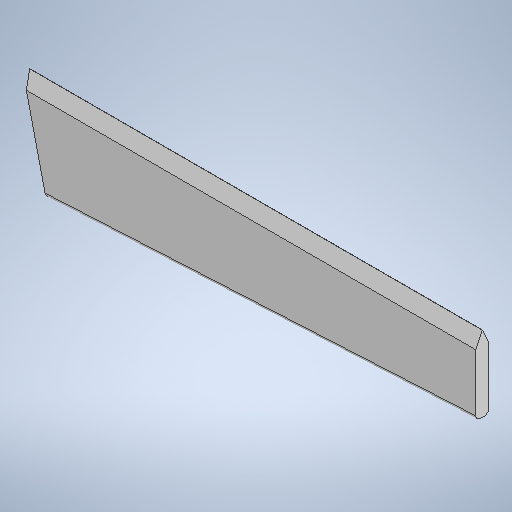
# Autodesk Inventor part: Part12
Saved by Autodesk Inventor 2025.3 (Build 293356000, 356)
## iProperties
Created: 2025-07-09
Part Number: Part12
Material: Generic
Document SubType Name: Modeling
Designer: steve
Density: 1 g/cm^3
Appearance: Default
Author: steve
Autodesk Inventor part; units mm, degrees
ref_plane "YZ Plane" through (0, 0, 0) normal (1, 0, 0) x (0, 1, 0)
ref_plane "XZ Plane" through (0, 0, 0) normal (0, 1, 0) x (-1, 0, 0)
ref_plane "XY Plane" through (0, 0, 0) normal (0, 0, 1) x (1, 0, 0)
sketch "Sketch1" plane through (0, 0, 0) normal (0, 0, 1) x (1, 0, 0)
  line L0 (-22.943, -21.4569) -> (193.057, -21.4569)
  line L1 (-22.943, -21.4569) -> (-12.943, -21.4569)
  line L2 (-12.943, -21.4569) -> (-2.943, -21.4569)
  line L3 (-2.943, -21.4569) -> (-2.943, -64.1369)
  line L4 (-22.943, -21.4569) -> (184.057, -21.4569)
  line L5 (184.057, -21.4569) -> (184.057, -54.3769)
  line L6 (184.057, -54.3769) -> (-2.943, -64.1369)
  line L7 (-12.943, -21.4569) -> (-2.943, -64.1369)
  line L8 (184.057, -21.4569) -> (184.057, 33.1531)
  line L9 (-22.943, -21.4569) -> (-22.943, 89.8331)
  line L10 (-22.943, 89.8331) -> (184.057, 33.1531)
  line L11 (184.057, 33.1531) -> (184.057, 34.1531)
  line L12 (184.057, 34.1531) -> (193.057, 31.6888)
  line L13 (193.057, -21.4569) -> (193.057, 31.6888)
  line L14 (184.057, -54.3769) -> (193.057, -53.9072)
  line L15 (193.057, -21.4569) -> (193.057, -53.9072)
  line L16 (-22.943, -21.4569) -> (-32.943, -21.4569)
  line L17 (-32.943, -21.4569) -> (-42.943, -21.4569)
  line L18 (-22.943, -21.4569) -> (-229.943, -21.4569)
  line L19 (-229.943, -21.4569) -> (-229.943, -54.3769)
  line L20 (-42.943, -21.4569) -> (-42.943, -64.1369)
  line L21 (-229.943, -54.3769) -> (-42.943, -64.1369)
  line L22 (-32.943, -21.4569) -> (-42.943, -64.1369)
  line L23 (-238.943, -21.4569) -> (-238.943, -53.9072)
  line L24 (-229.943, -54.3769) -> (-238.943, -53.9072)
  line L25 (-22.943, -21.4569) -> (-238.943, -21.4569)
  line L26 (-238.943, -21.4569) -> (-238.943, 31.6888)
  line L27 (-229.943, 34.1531) -> (-238.943, 31.6888)
  line L28 (-229.943, -21.4569) -> (-229.943, 33.1531)
  line L29 (-229.943, 33.1531) -> (-229.943, 34.1531)
  line L30 (-22.943, 89.8331) -> (-229.943, 33.1531)
  point P0 (0, 0)
  dimension "d0" = 216
  dimension "d1" = 10
  dimension "d2" = 10
  dimension "d3" = 42.68
  dimension "d4" = 207
  dimension "d5" = 32.92
  dimension "d6" = 54.61
  dimension "d7" = 111.29
  dimension "d8" = 1
  constraints: 62 end point, 10 symmetric about line, 7 vertical, 6 point on line, 1 collinear, 1 horizontal, 1 parallel
  measures "d0" distance of L9.start L15.start
  measures "d1" distance of L9.start L7.start
  measures "d2" distance of L7.start L3.start
  measures "d3" distance of L3.start L6.end
  measures "d4" distance of L9.start L5.start
  measures "d5" distance of L5.start L14.start
  measures "d6" distance of L5.start L8.end
  measures "d7" distance of L9.start L9.end
  measures "d8" distance of L8.end L11.end
extrude "Extrusion1" add sketch "Sketch1" along normal mid plane 5.7 contours L0 L3 L7 | L0 L5 L6 L3
chamfer "Chamfer1" distance 6 angle 25 1 edges at (85.557, -21.4569, -2.85) measured on face at (56.057, -35.6836, -2.85)
fillet "Fillet1" radius 2 1 edges at (90.557, -59.2569, 2.85)
fillet "Fillet2" radius 2 1 edges at (90.557, -59.2569, -2.85)
chamfer "Chamfer2" distance 6 angle 25 1 edges at (85.557, -21.4569, 2.85) measured on face at (55.9024, -35.0241, 2.85)
body "Solid1"
